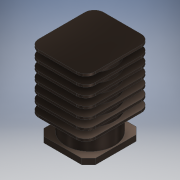
# Autodesk Inventor part: Part2
Saved by Autodesk Inventor 2019 (Build 230136000, 136)
## iProperties
Created: 2022-01-28
Part Number: Part2
Material: Generic
Document SubType Name: Modeling
Designer: Sepehr
Density: 1 g/cm^3
Appearance: Default
Author: Sepehr
Autodesk Inventor part; units mm, degrees
ref_plane "YZ Plane" through (0, 0, 0) normal (1, 0, 0) x (0, 1, 0)
ref_plane "XZ Plane" through (0, 0, 0) normal (0, 1, 0) x (-1, 0, 0)
ref_plane "XY Plane" through (0, 0, 0) normal (0, 0, 1) x (1, 0, 0)
sketch "Sketch1" plane through (0, 0, 0) normal (0, 1, 0) x (-1, 0, 0)
  line L0 (2900, -2000) -> (2900, 2000)
  line L1 (-2900, 2000) -> (-2900, -2000)
  line L2 (0, -2750) -> (-2150, -2750)
  line L3 (-2150, -2750) -> (2150, -2750)
  line L4 (0, 2750) -> (-2150, 2750)
  line L5 (-2150, 2750) -> (2150, 2750)
  line L6 (2150, -2750) -> (2900, -2000)
  line L7 (-2150, -2750) -> (-2900, -2000)
  line L8 (-2900, 2000) -> (-2150, 2750)
  line L9 (2150, 2750) -> (2900, 2000)
  point P0 (2900, -2750)
  point P1 (2900, 2750)
  constraints: 20 end point, 2 point on line, 1 parallel
extrude "Extrusion1" add sketch "Sketch1" along normal blind 600
sketch "Sketch2" plane through (0, 600, 0) normal (0, 1, 0) x (1, 0, 0)
  circle A0 centre (0, 0) radius 2600
  constraints: 1 centre point
extrude "Extrusion2" add sketch "Sketch2" along normal blind 8000
sketch "Sketch4" plane through (0, 8600, 0) normal (0, 1, 0) x (1, 0, 0)
  line L0 (2450, 3000) -> (-2450, 3000)
  line L1 (-3450, 2000) -> (-3450, -2000)
  line L2 (-2450, -3000) -> (2450, -3000)
  line L3 (3450, -2000) -> (3450, 2000)
  arc A0 (-2450, 3000) -> (-3450, 2000) centre (-2450, 2000) ccw
  arc A1 (3450, 2000) -> (2450, 3000) centre (2450, 2000) ccw
  arc A2 (2450, -3000) -> (3450, -2000) centre (2450, -2000) ccw
  arc A3 (-3450, -2000) -> (-2450, -3000) centre (-2450, -2000) ccw
  constraints: 8 end point, 8 point on circle, 8 tangent, 4 centre point, 3 equal radius, 2 parallel, 1 horizontal, 1 perpendicular
extrude "Extrusion3" add sketch "Sketch4" along normal blind 250
pattern_linear "Rectangular Pattern1" count 7 spacing 1000 along (0, -1, 0) of "Extrusion3"
sketch "Sketch5" plane through (0, 0, 0) normal (0, -1, 0) x (1, 0, 0)
  circle A0 centre (0, 0) radius 2350
  dimension "d29" = 4700
  constraints: 1 centre point, 1 coincident
  measures "d29" diameter of A0
extrude "Extrusion4" cut sketch "Sketch5" against normal blind 8600
body "Solid1"
